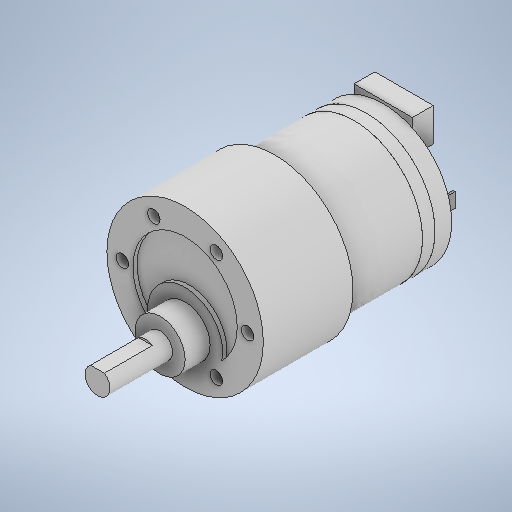
# Autodesk Inventor part: 520 DC Gear Motor
Saved by Autodesk Inventor 2025.2 (Build 292293000, 293)
## iProperties
Created: 2025-01-16
Part Number: 520 DC Gear Motor
Material: Generic
Document SubType Name: Modeling
Designer: Matt Tidd
Density: 1 g/cm^3
Appearance: Default
Author: Matt Tidd
Autodesk Inventor part; units mm, degrees
ref_plane "YZ Plane" through (0, 0, 0) normal (1, 0, 0) x (0, 1, 0)
ref_plane "XZ Plane" through (0, 0, 0) normal (0, 1, 0) x (-1, 0, 0)
ref_plane "XY Plane" through (0, 0, 0) normal (0, 0, 1) x (1, 0, 0)
sketch "Sketch1" plane through (0, 0, 0) normal (0, 0, 1) x (1, 0, 0)
  circle A0 centre (0, 0) radius 18.75
  dimension "d0" = 37.5
  constraints: 1 centre point, 1 coincident
  measures "d0" diameter of A0
extrude "Extrusion1" add sketch "Sketch1" along normal blind 21.5
sketch "Sketch2" plane through (0, 0, 0) normal (0, 0, -1) x (-1, 0, 0)
  circle A0 centre (0, 0) radius 16.4
  dimension "d3" = 32.8
  constraints: 1 centre point, 1 coincident
  measures "d3" diameter of A0
extrude "Extrusion2" add sketch "Sketch2" along normal blind 19
sketch "Sketch3" plane through (0, 0, 21.5) normal (0, 0, 1) x (1, 0, 0)
  circle A0 centre (0, -7) radius 6
  point P0 (0, 0)
  dimension "d6" = 12
  constraints: 1 centre point
  measures "d6" diameter of A0
extrude "Extrusion3" add sketch "Sketch3" along normal blind 6
sketch "Sketch4" plane through (0, -7, 27.5) normal (0, 0, 1) x (1, 0, 0)
  circle A0 centre (0, 0) radius 6 projected
  circle A1 centre (0, 0) radius 3
  point P0 (0, 7)
  dimension "d9" = 6
  constraints: 1 centre point, 1 coincident
  measures "d9" diameter of A1
extrude "Extrusion4" add sketch "Sketch4" along normal blind 15 contours A1
sketch "Sketch5" plane through (0, -7, 42.5) normal (0, 0, 1) x (1, 0, 0)
  line L0 (0, 2.5) -> (1.6583, 2.5)
  line L1 (1.6583, 2.5) -> (-1.6583, 2.5)
  circle A0 centre (0, 0) radius 3 projected
  point P0 (0, 7)
  constraints: 4 end point, 2 point on circle, 1 horizontal
extrude "Extrusion5" cut sketch "Sketch5" against normal blind 11.5 contours L1 A0 L0 picked at (-0.897, 2.6056)
sketch "Sketch6" plane through (0, 0, 21.5) normal (0, 0, 1) x (1, 0, 0)
  circle A0 centre (0, 0) radius 15 construction
  circle A1 centre (15, 0) radius 1.5
  circle A2 centre (7.5, 12.9904) radius 1.5
  circle A3 centre (-7.5, 12.9904) radius 1.5
  circle A4 centre (-15, 0) radius 1.5
  circle A5 centre (-7.5, -12.9904) radius 1.5
  circle A6 centre (7.5, -12.9904) radius 1.5
  dimension "d14" = 30
  dimension "d15" = 3
  dimension "d18" = 360
  constraints: 6 centre point, 1 coincident, 1 horizontal alignment, 15 other
  measures "d15" diameter of A1
extrude "Extrusion6" cut sketch "Sketch6" against normal blind 5
sketch "Sketch7" plane through (0, 0, -19) normal (0, 0, -1) x (-1, 0, 0)
  circle A0 centre (0, 0) radius 16.4
  constraints: 1 centre point, 1 coincident
extrude "Extrusion7" add sketch "Sketch7" along normal blind 3 separate body
sketch "Sketch8" plane through (0, 0, -22) normal (0, 0, -1) x (-1, 0, 0)
  circle A0 centre (0, 0) radius 16.4
  constraints: 1 centre point, 1 coincident
extrude "Extrusion8" add sketch "Sketch8" along normal blind 4 separate body
sketch "Sketch9" plane through (0, 0, -26) normal (0, 0, -1) x (-1, 0, 0)
  circle A0 centre (0, 0) radius 6.5
  dimension "d26" = 13
  constraints: 1 centre point, 1 coincident
  measures "d26" diameter of A0
extrude "Extrusion9" add sketch "Sketch9" along normal blind 6.5 separate body
sketch "Sketch10" plane through (0, 0, -32.5) normal (0, 0, -1) x (-1, 0, 0)
  circle A0 centre (0, 0) radius 0.5
  dimension "d29" = 1
  constraints: 1 centre point, 1 coincident
  measures "d29" diameter of A0
extrude "Extrusion10" add sketch "Sketch10" along normal blind 1 separate body
sketch "Sketch11" plane through (0, 0, 21.5) normal (0, 0, 1) x (1, 0, 0)
  circle A0 centre (0, 0) radius 0.5 projected
  circle A1 centre (0, 0) radius 12.5
  circle A2 centre (0, -7) radius 6 projected
  circle A3 centre (0, -7) radius 9
  point P0 (-8.8025, -8.875)
  point P1 (8.8025, -8.875)
  dimension "d32" = 25
  dimension "d33" = 18
  constraints: 2 centre point, 2 coincident
  measures "d32" diameter of A1
  measures "d33" diameter of A3
extrude "Extrusion11" cut sketch "Sketch11" against normal blind 1 contours A1 A3 bodies 1
sketch "Sketch12" plane through (0, 0, -26) normal (0, 0, -1) x (-1, 0, 0)
  line L0 (0, 9) -> (14.8265, 9) construction
  line L1 (14.8265, 9) -> (-13.5735, 9) construction
  line L2 (0, 9) -> (7, 9)
  line L3 (7, 9) -> (7, 17)
  line L4 (7, 17) -> (0, 17)
  line L5 (0, 17) -> (0, 9)
  line L6 (0, 17) -> (-7, 17)
  line L7 (-7, 17) -> (-7, 9)
  line L8 (-7, 9) -> (0, 9)
  line L9 (0, 9) -> (0, 17)
  point P0 (0, 0)
  dimension "d36" = 7
  dimension "d37" = 8
  dimension "d38" = 7
  constraints: 20 end point, 4 parallel, 3 horizontal, 2 perpendicular, 2 point on line
  measures "d36" distance of L4.end L3.end
  measures "d37" distance of L3.end L2.end
  measures "d38" distance of L8.end L7.end
extrude "Extrusion12" add sketch "Sketch12" along normal blind 5 bodies 3
sketch "Sketch13" plane through (0, 0, -26) normal (0, 0, -1) x (-1, 0, 0)
  circle A0 centre (0, 0) radius 0.5 projected
  line L0 (0, 0) -> (11.75, 0)
  line L1 (11.75, 0) -> (11.75, 1.75)
  line L2 (11.75, 1.75) -> (12.25, 1.75)
  line L3 (12.25, 1.75) -> (12.25, -1.75)
  line L4 (12.25, -1.75) -> (11.75, -1.75)
  line L5 (11.75, -1.75) -> (11.75, 1.75)
  line L6 (0, 0) -> (0, 8.55) construction
  line L7 (0, 0) -> (-11.75, 0)
  line L8 (-11.75, 0) -> (-11.75, 1.75)
  line L9 (-11.75, 1.75) -> (-12.25, 1.75)
  line L10 (-12.25, 1.75) -> (-12.25, -1.75)
  line L11 (-12.25, -1.75) -> (-11.75, -1.75)
  line L12 (-11.75, -1.75) -> (-11.75, 1.75)
  dimension "d41" = 11.75
  dimension "d42" = 1.75
  dimension "d43" = 0.5
  dimension "d44" = 3.5
  constraints: 26 end point, 5 symmetric about line, 2 horizontal, 2 parallel, 2 vertical, 1 perpendicular
  measures "d41" distance of L0.start L0.end
  measures "d42" distance of L0.end L1.end
  measures "d43" distance of L3.end L4.end
  measures "d44" distance of L2.end L3.end
extrude "Extrusion13" add sketch "Sketch13" along normal blind 5 contours L1 L2 L3 L4 L5 | L12 L11 L10 L9 L8 bodies 3
body "Solid1"
body "Solid2"
body "Solid3"
body "Solid4"
body "Solid5"
